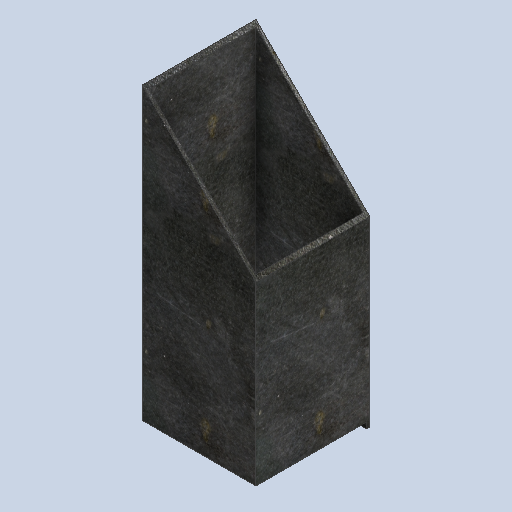
# Autodesk Inventor part: WI-ShaftRS3
Saved by Autodesk Inventor 2024.3 (Build 283343000, 343)
## iProperties
Created: 2025-06-13
Part Number: WI-ShaftRS3
Material: Steel
Document SubType Name: Modeling
Designer: ajclo
Density: 7.85 g/cm^3
Appearance: Plate
Mass: 1874.34 g
Surface Area: 1620.2 cm^2
Volume: 238.77 cm^3
Author: ajclo
Autodesk Inventor part; units mm, degrees
ref_plane "YZ Plane" through (0, 0, 0) normal (1, 0, 0) x (0, 1, 0)
ref_plane "XZ Plane" through (0, 0, 0) normal (0, 1, 0) x (-1, 0, 0)
ref_plane "XY Plane" through (0, 0, 0) normal (0, 0, 1) x (1, 0, 0)
sketch "Sketch1" plane through (0, 0, 0) normal (0, 1, 0) x (-1, 0, 0)
  line L0 (50, 50) -> (-50, 50)
  line L1 (-50, 50) -> (-50, -50)
  line L2 (-50, -50) -> (50, -50)
  line L3 (50, -50) -> (50, 50)
  line L4 (50, 50) -> (-50, -50) construction
  line L5 (-50, 50) -> (50, -50) construction
  line L6 (47, 47) -> (-47, 47)
  line L7 (-47, 47) -> (-47, -47)
  line L8 (-47, -47) -> (47, -47)
  line L9 (47, -47) -> (47, 47)
  line L10 (47, 47) -> (-47, -47) construction
  line L11 (-47, 47) -> (47, -47) construction
  point P0 (0, 0)
  dimension "d0" = 3
  dimension "d1" = 3
  dimension "d2" = 100
  dimension "d3" = 100
  constraints: 24 end point, 4 midpoint, 4 parallel, 2 horizontal, 2 perpendicular
  measures "d0" distance between parallel lines of L3 L9
  measures "d1" distance between parallel lines of L2 L8
  measures "d2" distance of L2.end L0.start
  measures "d3" distance of L1.end L2.end
extrude "Extrusion1" add sketch "Sketch1" along normal blind 255
sketch "Sketch2" plane through (-50, 0, 50) normal (0, 0, 1) x (1, 0, 0)
  line L0 (0, 0) -> (100, 0) projected
  line L1 (100, 0) -> (100, 255) projected
  line L2 (0, 255) -> (100, 255) projected
  line L3 (0, 0) -> (0, 255) projected
  line L4 (0, 255) -> (100, 155)
  point P0 (50, 0)
  dimension "d6" = 45
  constraints: 2 end point, 1 point on line
  measures "d6" angle of L2 L4
extrude "Extrusion2" cut sketch "Sketch2" against normal through all contours L2 L1 L4
sketch "Sketch3" plane through (0, 0, 0) normal (0, -1, 0) x (1, 0, 0)
  line L0 (-47, -47) -> (-47, 47) projected
  line L1 (-50, -50) -> (-50, 50) projected
  line L2 (-47, 25) -> (-50, 25)
  line L3 (-50, 25) -> (-50, 22)
  line L4 (-50, 22) -> (-47, 22)
  line L5 (-47, 22) -> (-47, 25)
  line L6 (50, -50) -> (50, 50) projected
  line L7 (50, -47) -> (40, -47)
  line L8 (40, -47) -> (40, -50)
  line L9 (40, -50) -> (50, -50)
  line L10 (50, -50) -> (50, -47)
  line L11 (50, 50) -> (50, -50) projected
  line L12 (-50, 50) -> (50, 50) projected
  line L13 (-50, -50) -> (-50, 50) projected
  line L14 (50, -50) -> (-50, -50) projected
  line L15 (-47, 47) -> (-47, -47) projected
  line L16 (47, 47) -> (-47, 47) projected
  line L17 (47, -47) -> (47, 47) projected
  line L18 (-47, -47) -> (47, -47) projected
  line L19 (50, -50) -> (-50, -50) projected
  point P0 (0, 0)
  point P1 (-48.5, 25)
  dimension "d9" = 10
  dimension "d10" = 3
  dimension "d11" = 25
  constraints: 16 end point, 4 parallel, 3 point on line, 2 collinear, 2 horizontal, 2 perpendicular, 1 midpoint
  measures "d9" distance between parallel lines of L6 L8
  measures "d10" distance between parallel lines of L2 L4
  measures "d11" distance from line of L12 point (-48.5, 25)
extrude "Extrusion3" add sketch "Sketch3" along normal blind 5 contours L7 L6 L9 L8
body "Solid1"
